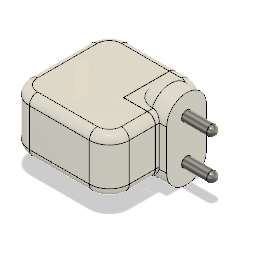
08-Day1 - iPhone Charging Adapter v2 (Autodesk Fusion 360 design; units mm, degrees)
Autodesk Fusion 360 part; units mm, degrees
sketch "Sketch1" plane through (0, 0, 0) normal (0, 1, 0) x (1, 0, 0)
  line L0 (-15, 25) -> (15, 25)
  line L1 (25, 15) -> (25, -15)
  line L2 (15, -25) -> (-15, -25)
  line L3 (-25, -15) -> (-25, 15)
  arc A0 (-15, 25) -> (-25, 15) centre (-15, 15) ccw
  arc A1 (25, 15) -> (15, 25) centre (15, 15) ccw
  arc A2 (15, -25) -> (25, -15) centre (15, -15) ccw
  arc A3 (-25, -15) -> (-15, -25) centre (-15, -15) ccw
  dimension "d1" = 10
  constraint horizontal L0
  constraint perpendicular L0 L1
  constraint parallel L0 L2
  constraint parallel L1 L3
  constraint tangent L0 A0
  constraint tangent L3 A0
  constraint tangent L0 A1
  constraint tangent L1 A1
  constraint equal A0 A1
  constraint tangent L1 A2
  constraint tangent L2 A2
  constraint equal A0 A2
  constraint tangent L2 A3
  constraint tangent L3 A3
  constraint equal A0 A3
  measures "d1" radius of A0
extrude "Extrude1" add sketch "Sketch1" along normal mid plane 28 makes body 1
sketch "Sketch2" plane through (0, 0, 0) normal (0, 1, 0) x (1, 0, 0)
  arc A0 (-15, 25) -> (-25, 15) centre (-15, 15) ccw
  line L0 (-25, 15) -> (-25, -15)
  arc A1 (-25, -15) -> (-15, -25) centre (-15, -15) ccw
  line L1 (-15, -25) -> (15, -25)
  arc A2 (15, -25) -> (25, -15) centre (15, -15) ccw
  line L2 (25, -15) -> (25, 15)
  arc A3 (25, 15) -> (15, 25) centre (15, 15) ccw
  line L3 (15, 25) -> (-15, 25)
  line L4 (23.6603, 20) -> (28.6603, 20)
  line L5 (23.6603, 20) -> (20.6603, 20)
  line L6 (28.6603, 20) -> (28.6603, 0)
  line L7 (10.6603, 10) -> (10.6603, 10)
  line L8 (20.6603, 0) -> (28.6603, 0)
  arc A4 (20.6603, 20) -> (10.6603, 10) centre (20.6603, 10) ccw
  arc A5 (10.6603, 10) -> (20.6603, 0) centre (20.6603, 10) ccw
  point P0 (10.6603, 20)
  dimension "d4" = 5
  dimension "d5" = 13
  dimension "d6" = 10
  constraint coincident A3 L4.start
  constraint perpendicular L4 L6
  constraint perpendicular L2 L8
  constraint coincident P0 L5
  constraint tangent L5 A4
  constraint tangent L8 A5
  constraint equal A4 A5
  measures "d4" distance of L4.start L4.end
  measures "d5" distance of L4.start P0
  measures "d6" radius of A4
extrude "Extrude4" add sketch "Sketch2" along normal mid plane 40 separate body contours L2 A3 L4 L6 L8 | L2 A3 L5 L8 A4 A5 makes body 2
fillet "Fillet3" radius 10 6 edges at (24.6603, -20, 0) (10.6603, -20, -10) (24.6603, -20, -20) (24.6603, 20, -20) (10.6603, 20, -10) (24.6603, 20, 0) on bodies 2
sketch "Sketch5" plane through (28.6603, 0, 0) normal (1, 0, 0) x (0, 0, -1)
  arc A0 (20, 10) -> (0, 10) centre (10, 10) ccw
  line L0 (0, 10) -> (0, -10)
  arc A1 (0, -10) -> (20, -10) centre (10, -10) ccw
  line L1 (20, -10) -> (20, 10)
  line L2 (10, 20) -> (10, 10)
  line L3 (10, -20) -> (10, -10)
  circle A2 centre (10, 10) radius 2.5
  circle A3 centre (10, -10) radius 2.5
  dimension "d19" = 5
  dimension "d20" = 5
  constraint midpoint A0 L2.start
  constraint coincident A0.centre L2.end
  constraint midpoint A1 L3.start
  constraint coincident A1.centre L3.end
  constraint concentric A0 A2
  measures "d19" diameter of A2
  measures "d20" diameter of A3
extrude "Extrude5" add sketch "Sketch5" along normal blind 15 separate body contours A2 | A3 makes body 3 at (38.6603, 10.2489, -12.4876) makes body 4 at (38.6603, -9.7511, -12.4876)
fillet "Fillet4" radius 2.5 2 edges at (43.6603, 9.096, -7.6692) (43.6603, -10.904, -7.6692) on bodies 3 4
sketch "Sketch6" plane through (-25, 0, 0) normal (-1, 0, 0) x (0, 0, 1)
  line L0 (15, -14) -> (15, 14)
  line L1 (15, 14) -> (-15, 14)
  line L2 (-15, 14) -> (-15, -14)
  line L3 (-15, -14) -> (15, -14)
  line L4 (-6, -7) -> (-12, -7)
  line L5 (-13, -6) -> (-13, 7)
  line L6 (-12, 8) -> (-6, 8)
  line L7 (-5, 7) -> (-5, -6)
  arc A0 (-12, 8) -> (-13, 7) centre (-12, 7) ccw
  arc A1 (-5, 7) -> (-6, 8) centre (-6, 7) ccw
  arc A2 (-6, -7) -> (-5, -6) centre (-6, -6) ccw
  arc A3 (-13, -6) -> (-12, -7) centre (-12, -6) ccw
  arc A4 (-12, 7.5) -> (-12.5, 7) centre (-12, 7) ccw
  line L8 (-12.5, -6) -> (-12.5, 7)
  arc A5 (-12.5, -6) -> (-12, -6.5) centre (-12, -6) ccw
  line L9 (-6, -6.5) -> (-12, -6.5)
  arc A6 (-6, -6.5) -> (-5.5, -6) centre (-6, -6) ccw
  line L10 (-5.5, 7) -> (-5.5, -6)
  arc A7 (-5.5, 7) -> (-6, 7.5) centre (-6, 7) ccw
  line L11 (-12, 7.5) -> (-6, 7.5)
  arc A8 (-12, 7.9) -> (-12.9, 7) centre (-12, 7) ccw
  line L12 (-12.9, -6) -> (-12.9, 7)
  arc A9 (-12.9, -6) -> (-12, -6.9) centre (-12, -6) ccw
  line L13 (-6, -6.9) -> (-12, -6.9)
  arc A10 (-6, -6.9) -> (-5.1, -6) centre (-6, -6) ccw
  line L14 (-5.1, 7) -> (-5.1, -6)
  arc A11 (-5.1, 7) -> (-6, 7.9) centre (-6, 7) ccw
  line L15 (-12, 7.9) -> (-6, 7.9)
  dimension "d25" = 1
  dimension "d26" = 0.5
  dimension "d27" = 0.1
  constraint perpendicular L4 L7
  constraint tangent L5 A0
  constraint tangent L6 A0
  constraint tangent L6 A1
  constraint tangent L7 A1
  constraint equal A0 A1
  constraint tangent L4 A2
  constraint tangent L7 A2
  constraint equal A0 A2
  constraint tangent L4 A3
  constraint tangent L5 A3
  constraint equal A0 A3
  measures "d25" radius of A0
extrude "Extrude6" cut sketch "Sketch6" against normal blind 13 contours L4 L5 L6 L7 A0 A1 A2 A3 | A4 L8 A5 L9 A6 L10 A7 L11 bodies 1
sketch "Sketch7" plane through (-12, 0, 0) normal (-1, 0, 0) x (0, 0, 1)
  arc A0 (-12.5, -6) -> (-12, -6.5) centre (-12, -6) ccw
  line L0 (-12, -6.5) -> (-6, -6.5)
  arc A1 (-6, -6.5) -> (-5.5, -6) centre (-6, -6) ccw
  line L1 (-5.5, -6) -> (-5.5, 7)
  arc A2 (-5.5, 7) -> (-6, 7.5) centre (-6, 7) ccw
  line L2 (-6, 7.5) -> (-12, 7.5)
  arc A3 (-12, 7.5) -> (-12.5, 7) centre (-12, 7) ccw
  line L3 (-12.5, 7) -> (-12.5, -6)
  line L4 (-12.5, -6) -> (-12.5, 7)
  line L5 (-11.5, 6.5) -> (-9.5, 6.5)
  line L6 (-9.5, 6.5) -> (-9.5, -5.5)
  line L7 (-9.5, -5.5) -> (-11.5, -5.5)
  line L8 (-11.5, -5.5) -> (-11.5, 6.5)
  constraint horizontal L5
  constraint vertical L6
  constraint horizontal L7
  constraint vertical L8
extrude "Extrude7" add sketch "Sketch7" along normal blind 10 separate body contours L5 L6 L7 L8 makes body 5
sketch "Sketch8" plane through (0, 0, -9.5) normal (0, 0, 1) x (1, 0, 0)
  line L0 (-12, 6.5) -> (-22, 6.5)
  line L1 (-22, 6.5) -> (-22, -5.5)
  line L2 (-22, -5.5) -> (-12, -5.5)
  line L3 (-12, -5.5) -> (-12, 6.5)
  line L4 (-21, 5) -> (-12, 5)
  line L5 (-12, 5) -> (-12, 4)
  line L6 (-12, 4) -> (-21, 4)
  line L7 (-21, 4) -> (-21, 5)
  line L8 (-21, 2.5) -> (-12, 2.5)
  line L9 (-12, 2.5) -> (-12, 1.5)
  line L10 (-12, 1.5) -> (-21, 1.5)
  line L11 (-21, 1.5) -> (-21, 2.5)
  line L12 (-21, 0) -> (-12, 0)
  line L13 (-12, 0) -> (-12, -1)
  line L14 (-12, -1) -> (-21, -1)
  line L15 (-21, -1) -> (-21, 0)
  line L16 (-21, -2.5) -> (-12, -2.5)
  line L17 (-12, -2.5) -> (-12, -3.5)
  line L18 (-12, -3.5) -> (-21, -3.5)
  line L19 (-21, -3.5) -> (-21, -2.5)
  dimension "d32" = 1
  constraint horizontal L4
  constraint vertical L5
  constraint horizontal L6
  constraint vertical L7
  constraint horizontal L8
  constraint vertical L9
  constraint horizontal L10
  constraint vertical L11
  constraint coincident L3 L9.end
  constraint horizontal L12
  constraint vertical L13
  constraint horizontal L14
  constraint vertical L15
  constraint coincident L3 L13.end
  constraint horizontal L16
  constraint vertical L17
  constraint horizontal L18
  constraint vertical L19
  constraint coincident L3 L17.end
  measures "d32" distance of L4.start L6.end
extrude "Extrude8" add sketch "Sketch8" along normal blind 0.01 contours L3 L4 L5 L6 L7 | L3 L8 L9 L10 L11 | L3 L16 L17 L18 L19 | L3 L12 L13 L14 L15 bodies 5
chamfer "Chamfer1" distance 0.25 angle 45 8 edges at (-22, 0.5, -9.5) (-22, 0.5, -11.5) (-22, 6.5, -10.5) (-22, -5.5, -10.5) (-17, -5.5, -9.5) (-17, -5.5, -11.5) (-17, 6.5, -9.5) (-17, 6.5, -11.5) on bodies 5
sketch "Sketch9" plane through (0, 14, 0) normal (0, 1, 0) x (-1, 0, 0)
  arc A0 (15, -25) -> (25, -15) centre (15, -15) ccw
  line L0 (25, -15) -> (25, 15)
  arc A1 (25, 15) -> (15, 25) centre (15, 15) ccw
  line L1 (15, 25) -> (-15, 25)
  arc A2 (-15, 25) -> (-25, 15) centre (-15, 15) ccw
  line L2 (-25, 15) -> (-25, -15)
  arc A3 (-25, -15) -> (-15, -25) centre (-15, -15) ccw
  line L3 (-15, -25) -> (15, -25)
  line L4 (-9, 2) -> (-9, -25)
  line L5 (-9, 2) -> (-25, 2)
  line L6 (-9.1, 1.9) -> (-9.1, -25)
  line L7 (-9.1, 1.9) -> (-25, 1.9)
  line L8 (-9.1, -25) -> (-9, -25)
  line L9 (-25, 2) -> (-25, 1.9)
  dimension "d36" = 0.1
  constraint coincident L2 L5.end
  constraint perpendicular L3 L4
  constraint coincident L3 L4.end
  constraint perpendicular L2 L5
  constraint perpendicular L4 L8
extrude "Extrude9" cut sketch "Sketch9" against normal blind 39 contours L2 L3 L4 L5 L6 L7 L8 L9 bodies 1 makes body 6 at (9.1, 4.6667, -7.0667)
sketch "Sketch10" plane through (0, 0, 0) normal (0, 1, 0) x (1, 0, 0)
  line L0 (20, -5) -> (0, -5)
  line L1 (0, -5) -> (0, 20)
  line L2 (0, 20) -> (20, 20)
  line L3 (20, 20) -> (20, -5)
  constraint horizontal L0
  constraint vertical L1
  constraint horizontal L2
  constraint vertical L3
extrude "Extrude10" add sketch "Sketch10" along normal mid plane 20 bodies 1 3 4 2 6
combine "Combine1" operation add target body 1 tool bodies 5
fillet "Fillet5" radius 4 10 edges at (-3, 14, -25) (-22.0711, 14, -22.0711) (-25, 14, 0) (-22.0711, 14, 22.0711) (0, 14, 25) (22.0711, 14, 22.0711) (25, 14, 8.5) (20.4013, 14, -23.4158) (12.05, 14, -25) (25, 14, 0.5326) on bodies 1
fillet "Fillet6" radius 5 10 edges at (25, -14, 8.5) (22.0711, -14, 22.0711) (0, -14, 25) (-22.0711, -14, 22.0711) (-25, -14, 0) (-22.0711, -14, -22.0711) (-3, -14, -25) (12.05, -14, -25) (20.4013, -14, -23.4158) (25, -14, 0.5326) on bodies 1
sketch "Sketch11" plane through (-12, 0, 0) normal (-1, 0, 0) x (0, 0, 1)
  line L0 (-9.5, -1) -> (-9.5, -2.5)
  line L1 (-9.5, -2.5) -> (-9.49, -2.5)
  line L2 (-9.49, -2.5) -> (-9.49, -3.5)
  line L3 (-9.49, -3.5) -> (-9.5, -3.5)
  line L4 (-9.5, -3.5) -> (-9.5, -5.25)
  line L5 (-9.5, -5.25) -> (-9.75, -5.5)
  line L6 (-9.75, -5.5) -> (-11.25, -5.5)
  line L7 (-11.25, -5.5) -> (-11.5, -5.25)
  line L8 (-11.5, -5.25) -> (-11.5, 6.25)
  line L9 (-11.5, 6.25) -> (-11.25, 6.5)
  line L10 (-11.25, 6.5) -> (-9.75, 6.5)
  line L11 (-9.75, 6.5) -> (-9.5, 6.25)
  line L12 (-9.5, 6.25) -> (-9.5, 5)
  line L13 (-9.5, 5) -> (-9.49, 5)
  line L14 (-9.49, 5) -> (-9.49, 4)
  line L15 (-9.49, 4) -> (-9.5, 4)
  line L16 (-9.5, 4) -> (-9.5, 2.5)
  line L17 (-9.5, 2.5) -> (-9.49, 2.5)
  line L18 (-9.49, 2.5) -> (-9.49, 1.5)
  line L19 (-9.49, 1.5) -> (-9.5, 1.5)
  line L20 (-9.5, 1.5) -> (-9.5, 0)
  line L21 (-9.5, 0) -> (-9.49, 0)
  line L22 (-9.49, 0) -> (-9.49, -1)
  line L23 (-9.49, -1) -> (-9.5, -1)
  arc A0 (-12.5, -6) -> (-12, -6.5) centre (-12, -6) ccw
  line L24 (-12, -6.5) -> (-6, -6.5)
  arc A1 (-6, -6.5) -> (-5.5, -6) centre (-6, -6) ccw
  line L25 (-5.5, -6) -> (-5.5, 7)
  arc A2 (-5.5, 7) -> (-6, 7.5) centre (-6, 7) ccw
  line L26 (-6, 7.5) -> (-12, 7.5)
  arc A3 (-12, 7.5) -> (-12.5, 7) centre (-12, 7) ccw
  line L27 (-12.5, 7) -> (-12.5, -6)
  line L28 (-12, 7.5) -> (-6, 7.5)
  line L29 (-5.5, 7) -> (-5.5, -6)
  line L30 (-12, -6.4) -> (-6, -6.4)
  arc A4 (-6, -6.4) -> (-5.6, -6) centre (-6, -6) ccw
  line L31 (-5.6, -6) -> (-5.6, 7)
  arc A5 (-5.6, 7) -> (-6, 7.4) centre (-6, 7) ccw
  line L32 (-6, 7.4) -> (-12, 7.4)
  arc A6 (-12, 7.4) -> (-12.4, 7) centre (-12, 7) ccw
  line L33 (-12.4, 7) -> (-12.4, -6)
  arc A7 (-12.4, -6) -> (-12, -6.4) centre (-12, -6) ccw
  dimension "d45" = -0.1
extrude "Extrude11" add sketch "Sketch11" along normal blind 11 contours A0 L24 A1 L25 A2 L26 A3 L27 L28 L29 bodies 1
